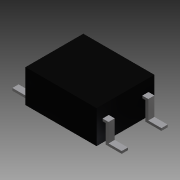
# Autodesk Inventor part: sTLP152 Optocoupler
Saved by Autodesk Inventor 2015 (Build 190159000, 159)
## iProperties
Created: 2016-01-19
Part Number: sTLP152 Optocoupler
Material: Generic
Document SubType Name: Modeling
Designer: Kyle
Density: 1 g/cm^3
Appearance: Default
Author: Kyle
Autodesk Inventor part; units mm, degrees
ref_plane "YZ Plane" through (0, 0, 0) normal (1, 0, 0) x (0, 1, 0)
ref_plane "XZ Plane" through (0, 0, 0) normal (0, 1, 0) x (-1, 0, 0)
ref_plane "XY Plane" through (0, 0, 0) normal (0, 0, 1) x (1, 0, 0)
sketch "Sketch1" plane through (0, 0, 0) normal (0, 0, 1) x (1, 0, 0)
  line L0 (0, 0) -> (4.5491, 0)
  line L1 (4.5491, 0) -> (4.5491, 2.1006)
  line L2 (4.5491, 2.1006) -> (0, 2.1006)
  line L3 (0, 2.1006) -> (0, 0)
  dimension "d0" = 2.1006
  dimension "d1" = 4.5491
  constraints: 8 end point, 2 parallel, 1 horizontal, 1 perpendicular
  measures "d0" distance of L0.end L1.end
  measures "d1" distance of L1.end L2.end
extrude "Extrusion1" add sketch "Sketch1" along normal blind 3.7008
sketch "Sketch2" plane through (4.5491, 0, 0) normal (1, 0, 0) x (0, 0, -1)
  line L0 (-3.3198, 1.3386) -> (-2.921, 1.3386)
  line L1 (-2.921, 1.3386) -> (-2.921, 1.1887)
  line L2 (-2.921, 1.1887) -> (-3.3198, 1.1887)
  line L3 (-3.3198, 1.1887) -> (-3.3198, 1.3386)
  line L4 (-0.7798, 1.3386) -> (-0.381, 1.3386)
  line L5 (-0.381, 1.3386) -> (-0.381, 1.1887)
  line L6 (-0.381, 1.1887) -> (-0.7798, 1.1887)
  line L7 (-0.7798, 1.1887) -> (-0.7798, 1.3386)
  line L8 (0, 0) -> (0, 2.1006) projected
  line L9 (0, 2.1006) -> (-3.7008, 2.1006) projected
  dimension "d4" = 0.3988
  dimension "d5" = 0.3988
  dimension "d6" = 0.1499
  dimension "d7" = 0.1499
  dimension "d8" = 2.1412
  dimension "d9" = 0
  dimension "d10" = 0.381
  dimension "d11" = 0.762
  constraints: 16 end point, 4 parallel, 2 horizontal, 2 perpendicular
  measures "d4" distance of L0.start L0.end
  measures "d5" distance of L4.start L4.end
  measures "d6" distance of L2.end L0.start
  measures "d7" distance of L4.end L5.end
  measures "d8" distance between parallel lines of L7 L1
  measures "d9" distance between parallel lines of L6 L2
  measures "d10" distance between parallel lines of L5 L8
  measures "d11" distance between parallel lines of L9 L0
extrude "Extrusion2" add sketch "Sketch2" against normal blind 4.7727
extrude "Extrusion3" add sketch "Sketch2" along normal blind 0.2286
sketch "Sketch3" plane through (4.7777, 0, 0) normal (1, 0, 0) x (0, 0, -1)
  line L0 (-3.3198, 1.3386) -> (-2.921, 1.3386)
  line L1 (-2.921, 1.3386) -> (-2.921, 1.1887)
  line L2 (-2.921, 1.1887) -> (-3.3198, 1.1887)
  line L3 (-3.3198, 1.1887) -> (-3.3198, 1.3386)
  line L4 (-0.7798, 1.3386) -> (-0.381, 1.3386)
  line L5 (-0.381, 1.3386) -> (-0.381, 1.1887)
  line L6 (-0.381, 1.1887) -> (-0.7798, 1.1887)
  line L7 (-0.7798, 1.1887) -> (-0.7798, 1.3386)
  point P0 (0, 0)
  constraints: 16 end point, 4 parallel, 2 horizontal, 2 perpendicular
extrude "Extrusion4" add sketch "Sketch3" along normal blind 0.1524
sketch "Sketch4" plane through (-0.2235, 0, 0) normal (-1, 0, 0) x (0, 0, 1)
  line L0 (2.921, 1.3386) -> (3.3198, 1.3386)
  line L1 (3.3198, 1.3386) -> (3.3198, 1.1887)
  line L2 (3.3198, 1.1887) -> (2.921, 1.1887)
  line L3 (2.921, 1.1887) -> (2.921, 1.3386)
  line L4 (0.381, 1.3386) -> (0.7798, 1.3386)
  line L5 (0.7798, 1.3386) -> (0.7798, 1.1887)
  line L6 (0.7798, 1.1887) -> (0.381, 1.1887)
  line L7 (0.381, 1.1887) -> (0.381, 1.3386)
  point P0 (0, 0)
  constraints: 16 end point, 4 parallel, 2 horizontal, 2 perpendicular
extrude "Extrusion5" add sketch "Sketch4" along normal blind 0.1524
sketch "Sketch5" plane through (0, 1.1887, 2.921) normal (0, -1, 0) x (1, 0, 0)
  line L0 (0, -2.1412) -> (-0.3759, -2.1412) projected
  line L1 (-0.3759, -2.54) -> (-0.188, -2.54)
  line L2 (-0.188, -2.54) -> (-0.188, -2.1412)
  line L3 (-0.188, -2.1412) -> (-0.3759, -2.1412)
  line L4 (-0.3759, -2.1412) -> (-0.3759, -2.54)
  line L5 (0, 0.3988) -> (-0.3759, 0.3988) projected
  line L6 (-0.3759, 0) -> (-0.188, 0)
  line L7 (-0.188, 0) -> (-0.188, 0.3988)
  line L8 (-0.188, 0.3988) -> (-0.3759, 0.3988)
  line L9 (-0.3759, 0.3988) -> (-0.3759, 0)
  line L10 (4.5491, -2.1412) -> (4.9301, -2.1412) projected
  line L11 (4.9301, -2.54) -> (4.7396, -2.54)
  line L12 (4.7396, -2.54) -> (4.7396, -2.1412)
  line L13 (4.7396, -2.1412) -> (4.9301, -2.1412)
  line L14 (4.9301, -2.1412) -> (4.9301, -2.54)
  line L15 (4.5491, 0.3988) -> (4.9301, 0.3988) projected
  line L16 (4.9301, 0) -> (4.7396, 0)
  line L17 (4.7396, 0) -> (4.7396, 0.3988)
  line L18 (4.7396, 0.3988) -> (4.9301, 0.3988)
  line L19 (4.9301, 0.3988) -> (4.9301, 0)
  point P0 (0, -2.921)
  constraints: 32 end point, 8 parallel, 4 horizontal, 4 midpoint, 4 perpendicular
extrude "Extrusion6" add sketch "Sketch5" along normal blind 1.1938
sketch "Sketch6" plane through (4.9301, 0, 0) normal (1, 0, 0) x (0, 0, -1)
  line L0 (-0.7798, 1.3386) -> (-0.7798, -0.0051) projected
  line L1 (-0.381, -0.0051) -> (-0.7798, -0.0051)
  line L2 (-0.7798, -0.0051) -> (-0.7798, 0.1473)
  line L3 (-0.7798, 0.1473) -> (-0.381, 0.1473)
  line L4 (-0.381, 0.1473) -> (-0.381, -0.0051)
  line L5 (-3.3198, 1.3386) -> (-3.3198, -0.0051) projected
  line L6 (-2.921, -0.0051) -> (-3.3198, -0.0051)
  line L7 (-3.3198, -0.0051) -> (-3.3198, 0.1473)
  line L8 (-3.3198, 0.1473) -> (-2.921, 0.1473)
  line L9 (-2.921, 0.1473) -> (-2.921, -0.0051)
  point P0 (0, 0)
  dimension "d22" = 0.1524
  constraints: 16 end point, 4 parallel, 2 horizontal, 2 perpendicular, 2 point on line
  measures "d22" distance between parallel lines of L1 L3
extrude "Extrusion7" add sketch "Sketch6" along normal blind 0.8433
sketch "Sketch7" plane through (-0.3759, 0, 0) normal (-1, 0, 0) x (0, 0, 1)
  line L0 (0.7798, -0.0051) -> (0.381, -0.0051)
  line L1 (0.381, -0.0051) -> (0.381, 0.1473)
  line L2 (0.381, 0.1473) -> (0.7798, 0.1473)
  line L3 (0.7798, 0.1473) -> (0.7798, -0.0051)
  line L4 (2.921, -0.0051) -> (3.3198, -0.0051)
  line L5 (3.3198, -0.0051) -> (3.3198, 0.1473)
  line L6 (3.3198, 0.1473) -> (2.921, 0.1473)
  line L7 (2.921, 0.1473) -> (2.921, -0.0051)
  point P0 (0, 0)
  constraints: 16 end point, 4 parallel, 2 horizontal, 2 perpendicular
extrude "Extrusion8" add sketch "Sketch7" along normal blind 0.8433
sketch "Sketch8" plane through (0, 1.1887, 0.7798) normal (0, 0, 1) x (1, 0, 0)
  line L0 (0, 0) -> (0, 0.1499)
  line L1 (0, 0.1499) -> (-0.3759, 0.1499)
  line L2 (0, 0.1499) -> (-0.3759, 0.1499) projected
  line L3 (-0.3759, 0.1499) -> (-0.3759, -1.0414)
  line L4 (-0.3759, -1.0414) -> (-1.2192, -1.0414)
  line L5 (-1.2192, -1.0414) -> (-1.2192, -1.1938)
  line L6 (-0.188, -1.1938) -> (-1.2192, -1.1938) projected
  line L7 (-1.2192, -1.1938) -> (-0.188, -1.1938)
  line L8 (-0.188, -1.1938) -> (-0.188, 0)
  line L9 (-0.188, 0) -> (0, 0)
  line L10 (0, 0) -> (-0.188, 0) projected
  point P0 (0, -1.1887)
  constraints: 16 end point, 5 perpendicular, 2 collinear, 1 vertical
extrude "Extrusion9" add sketch "Sketch8" along normal blind 1.27
extrude "Extrusion10" cut sketch "Sketch8" along normal blind 0.8712
body "Solid1"
